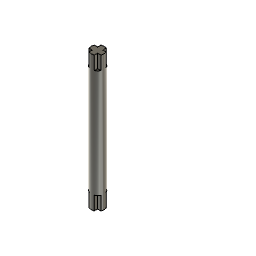
Bar (Autodesk Fusion 360 design; units mm, degrees)
Autodesk Fusion 360 part; units mm, degrees
sketch "Sketch1" plane through (0, 0, 0) normal (0, 0, 1) x (1, 0, 0)
  circle A0 centre (0, 0) radius 2.4
  dimension "d1" = 4.8
  constraint coincident A0.centre origin
  measures "d1" diameter of A0
extrude "Extrude1" add sketch "Sketch1" along normal blind 50
sketch "Sketch2" plane through (0, 0, 50) normal (0, 0, 1) x (-1, 0, 0)
  circle A0 centre (0, 0) radius 2.4
  line L0 (0.9817, -0.9817) -> (-0.9817, -0.9817)
  line L1 (-0.9817, -0.9817) -> (-0.9817, 0.9817)
  line L2 (-0.9817, 0.9817) -> (0.9817, 0.9817)
  line L3 (0.9817, 0.9817) -> (0.9817, -0.9817)
  line L4 (0.9817, -0.9817) -> (-0.9817, 0.9817) construction
  line L5 (-0.9817, -0.9817) -> (0.9817, 0.9817) construction
  line L6 (0.9817, -0.9817) -> (2.1901, -0.9817)
  line L7 (0.9817, 0.9817) -> (2.1901, 0.9817)
  line L8 (-0.9817, 0.9817) -> (-2.1901, 0.9817)
  line L9 (-0.9817, -0.9817) -> (-2.1901, -0.9817)
  line L10 (-0.9817, -0.9817) -> (-0.9817, -2.1901)
  line L11 (0.9817, -0.9817) -> (0.9817, -2.1901)
  line L12 (0.9817, 0.9817) -> (0.9817, 2.1901)
  line L13 (-0.9817, 0.9817) -> (-0.9817, 2.1901)
  constraint horizontal L0
  constraint perpendicular L0 L1
  constraint parallel L0 L2
  constraint parallel L1 L3
  constraint coincident L4 A0.centre
  constraint coincident L5 A0.centre
  constraint coincident A0.centre origin
  constraint coincident A0 L6.end
  constraint perpendicular L3 L6
  constraint coincident A0 L7.end
  constraint perpendicular L3 L7
  constraint coincident A0 L8.end
  constraint perpendicular L1 L8
  constraint coincident A0 L9.end
  constraint perpendicular L1 L9
  constraint coincident A0 L10.end
  constraint perpendicular L0 L10
  constraint coincident A0 L11.end
  constraint perpendicular L6 L11
  constraint coincident A0 L12.end
  constraint perpendicular L7 L12
  constraint coincident A0 L13.end
  constraint perpendicular L8 L13
extrude "Extrude2" cut sketch "Sketch2" against normal blind 5 contours A0 L7 L12 | A0 L6 L11 | A0 L8 L13 | A0 L9 L10
ref_plane "WorkPlane1" through (0, 0, 25) normal (0, 0, 1) x (1, 0, 0)
mirror "Mirror1" about plane through (0, 0, 25) normal (0, 0, 1) of "Extrude2"
